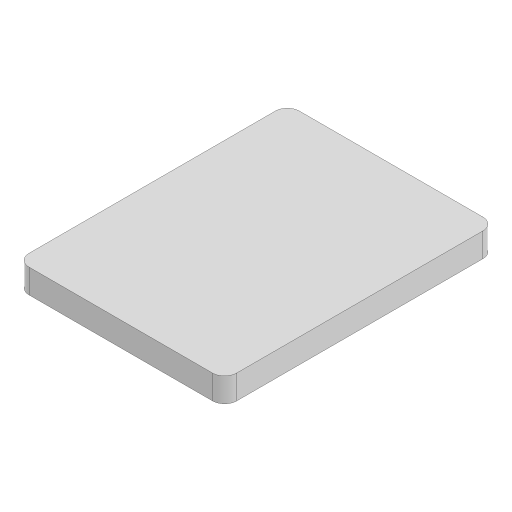
# Autodesk Inventor part: PLACA DE SOPORTE
Saved by Autodesk Inventor 2024 (Build 280153000, 153)
## iProperties
Created: 2024-05-16
Part Number: PLACA DE SOPORTE
Material: Generic
Document SubType Name: Modeling
Designer: Jhuliams
Density: 1 g/cm^3
Appearance: Default
Author: Jhuliams
Autodesk Inventor part; units mm, degrees
ref_plane "YZ Plane" through (0, 0, 0) normal (1, 0, 0) x (0, 1, 0)
ref_plane "XZ Plane" through (0, 0, 0) normal (0, 1, 0) x (-1, 0, 0)
ref_plane "XY Plane" through (0, 0, 0) normal (0, 0, 1) x (1, 0, 0)
sketch "Sketch1" plane through (0, 0, 0) normal (0, 1, 0) x (-1, 0, 0)
  line L0 (43, 56) -> (-43, 56)
  line L1 (-43, 56) -> (-43, -56)
  line L2 (-43, -56) -> (43, -56)
  line L3 (43, -56) -> (43, 56)
  line L4 (43, 56) -> (-43, -56) construction
  line L5 (-43, 56) -> (43, -56) construction
  point P0 (0, 0)
  dimension "d0" = 86
  dimension "d1" = 112
  constraints: 12 end point, 2 midpoint, 2 parallel, 1 horizontal, 1 perpendicular
  measures "d0" distance of L2.end L1.end
  measures "d1" distance of L1.end L0.end
extrude "Extrusion1" add sketch "Sketch1" along normal blind 10
fillet "Fillet1" radius 5 4 edges at (-43, 5, 56) (43, 5, 56) (43, 5, -56) (-43, 5, -56)
body "Solid1"
